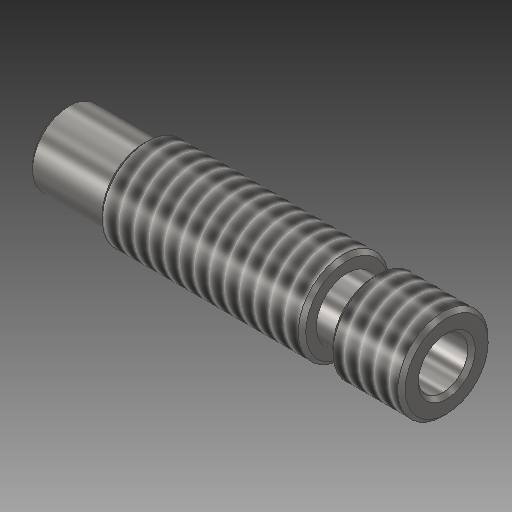
# Autodesk Inventor part: Vis de raccord
Saved by Autodesk Inventor 2017 (Build 210142000, 142)
## iProperties
Company: FABLAB Frenchmakers
Part Number: Vis de raccord
Material: Acier
Document SubType Name: Modeling
Designer: Adrien MARY
Density: 8 g/cm^3
Appearance: Semi-poli(2)
Mass: 3.33945 g
Surface Area: 7.62687 cm^2
Volume: 0.417431 cm^3
Project: 1420 Vauban 3D XL
Catalog Web Link: http://frenchmakers.com/
Stock Number: 1420-02-23
Autodesk Inventor part; units mm, degrees
ref_plane "YZ Plane" through (0, 0, 0) normal (1, 0, 0) x (0, 1, 0)
ref_plane "XZ Plane" through (0, 0, 0) normal (0, 1, 0) x (-1, 0, 0)
ref_plane "XY Plane" through (0, 0, 0) normal (0, 0, 1) x (1, 0, 0)
sketch "Esquisse1" plane through (0, 0, 0) normal (0, 0, 1) x (1, 0, 0)
  line L0 (0, 1.65) -> (0, 3)
  line L1 (0, 3) -> (-4.8, 3)
  line L2 (-4.8, 3) -> (-4.8, 2.05)
  line L3 (-4.8, 2.05) -> (-6.6, 2.05)
  line L4 (-6.6, 2.05) -> (-6.6, 3)
  line L5 (-6.6, 3) -> (-20.1, 3)
  line L6 (-20.1, 3) -> (-20.1, 2.425)
  line L7 (-20.1, 2.425) -> (-25.3, 2.425)
  line L8 (-25.3, 2.425) -> (-25.3, 1.65)
  line L9 (-25.3, 1.65) -> (0, 1.65)
  line L10 (0, 0) -> (-19.9979, 0)
  dimension "d0" = 6
  dimension "d1" = 3.3
  dimension "d2" = 4.1
  dimension "d3" = 4.8
  dimension "d4" = 13.5
  dimension "d5" = 1.8
  dimension "d6" = 4.85
  dimension "d7" = 25.3
  constraints: 22 end point, 6 perpendicular, 3 vertical, 1 collinear, 1 horizontal, 1 parallel, 1 vertical alignment
  measures "d0" diameter of L1 L10
  measures "d1" diameter of L9 L10
  measures "d2" diameter of L3 L10
  measures "d3" distance between parallel lines of L0 L2
  measures "d4" distance from line of L5.end L4
  measures "d5" distance between parallel lines of L4 L2
  measures "d6" diameter of L7 L10
  measures "d7" distance between parallel lines of L0 L8
revolve "Révolution1" add sketch "Esquisse1" angle 360 about axis through (0, 0, 0) along (-1, 0, 0)
chamfer "Chanfrein1" distance 0.25 angle 45 7 edges at (0, -1.65, 0) (0, -3, 0) (-25.3, -2.425, 0) (-25.3, -1.65, 0) (-4.8, -3, 0) (-6.6, -3, 0) (-20.1, -3, 0)
thread "Filetage1" size "M6x1" class "6g" standard "ANSI Metric M Profile" full length
thread "Filetage2" size "M6x1" class "6g" standard "ANSI Metric M Profile" full length
